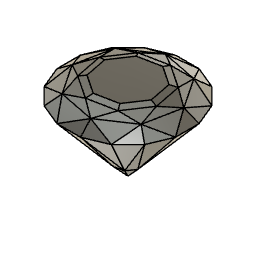
Diamond (Autodesk Fusion 360 design; units mm, degrees)
Autodesk Fusion 360 part; units mm, degrees
sketch "Sketch1" plane through (0, 0, 0) normal (0, 0, 1) x (1, 0, 0)
  line L0 (-3.5804, 18) -> (-10.1962, 15.2597)
  line L1 (-10.1962, 15.2597) -> (-15.2597, 10.1962)
  line L2 (-15.2597, 10.1962) -> (-18, 3.5804)
  line L3 (-18, 3.5804) -> (-18, -3.5804)
  line L4 (-18, -3.5804) -> (-15.2597, -10.1962)
  line L5 (-15.2597, -10.1962) -> (-10.1962, -15.2597)
  line L6 (-10.1962, -15.2597) -> (-3.5804, -18)
  line L7 (-3.5804, -18) -> (3.5804, -18)
  line L8 (3.5804, -18) -> (10.1962, -15.2597)
  line L9 (10.1962, -15.2597) -> (15.2597, -10.1962)
  line L10 (15.2597, -10.1962) -> (18, -3.5804)
  line L11 (18, -3.5804) -> (18, 3.5804)
  line L12 (18, 3.5804) -> (15.2597, 10.1962)
  line L13 (15.2597, 10.1962) -> (10.1962, 15.2597)
  line L14 (10.1962, 15.2597) -> (3.5804, 18)
  line L15 (3.5804, 18) -> (-3.5804, 18)
  dimension "d1" = 18
  measures "d1" distance of origin L15
extrude "Extrude1" add sketch "Sketch1" along normal blind 0 and the other way blind 17 draft -40
extrude "Extrude2" add 1 faces at (0.28, -1.4078, 0) along direction (0, 0, 1) blind 2.6 draft -56
sketch "Sketch2" plane through (0, 0, 2.6) normal (0, 0, 1) x (-1, 0, 0)
  line L0 (-8.0127, -11.9918) -> (-2.8137, -14.1453)
  line L1 (-2.8137, -14.1453) -> (2.8137, -14.1453)
  line L2 (2.8137, -14.1453) -> (8.0127, -11.9918)
  line L3 (8.0127, -11.9918) -> (11.9918, -8.0127)
  line L4 (11.9918, -8.0127) -> (14.1453, -2.8137)
  line L5 (14.1453, -2.8137) -> (14.1453, 2.8137)
  line L6 (14.1453, 2.8137) -> (11.9918, 8.0127)
  line L7 (11.9918, 8.0127) -> (8.0127, 11.9918)
  line L8 (8.0127, 11.9918) -> (2.8137, 14.1453)
  line L9 (2.8137, 14.1453) -> (-2.8137, 14.1453)
  line L10 (-2.8137, 14.1453) -> (-8.0127, 11.9918)
  line L11 (-8.0127, 11.9918) -> (-11.9918, 8.0127)
  line L12 (-11.9918, 8.0127) -> (-14.1453, 2.8137)
  line L13 (-14.1453, 2.8137) -> (-14.1453, -2.8137)
  line L14 (-14.1453, -2.8137) -> (-11.9918, -8.0127)
  line L15 (-11.9918, -8.0127) -> (-8.0127, -11.9918)
  line L16 (-2.8137, 14.1453) -> (-11.9918, 8.0127)
  line L17 (-10.1962, 15.2597, -2.6) -> (-2.8137, 14.1453, 0)
  line L18 (-10.1962, 15.2597, -2.6) -> (-11.9918, 8.0127, 0)
  point P0 (-10.1962, 15.2597)
  point P1 (-10.1962, 15.2597)
  constraint coincident L9.end L10.start
  constraint coincident L11.end L12.start
  constraint coincident P1 P0
extrude "Extrude3" cut sketch "Sketch2" along normal blind 1.5 contours L16 L17 L18 in plane through (1.5618, -2.3374, 8.0365) normal (0.255187, -0.381915, 0.888268)
pattern_circular "C-Pattern1" count 8 over 360 about axis through (0, 0, 1.75) along (0, 0, 1) of "Extrude3"
extrude "Extrude4" add 1 faces at (-0.9379, 4.7151, 2.6) along direction (0, 0, 1) blind 1.2 draft -62.7
sketch "Sketch3" plane through (0, 0, 3.8) normal (0, 0, 1) x (-1, 0, 0)
  line L0 (11.6772, 2.3227) -> (6.6146, 9.8994)
  line L1 (6.6146, 9.8994) -> (-2.3227, 11.6772)
  line L2 (-2.3227, 11.6772) -> (-9.8994, 6.6146)
  line L3 (-9.8994, 6.6146) -> (-11.6772, -2.3227)
  line L4 (-11.6772, -2.3227) -> (-6.6146, -9.8994)
  line L5 (-6.6146, -9.8994) -> (2.3227, -11.6772)
  line L6 (2.3227, -11.6772) -> (9.8994, -6.6146)
  line L7 (9.8994, -6.6146) -> (11.6772, 2.3227)
  line L8 (-6.1111, 9.1459) -> (-10.7883, 2.1459)
  line L9 (-10.7883, 2.1459, 0) -> (-11.9918, 8.0127, -1.2)
  line L10 (-11.9918, 8.0127, -1.2) -> (-6.1111, 9.1459, 0)
  point P0 (-11.9918, 8.0127)
  constraint midpoint L2 L8.start
  constraint midpoint L3 L8.end
extrude "Extrude5" cut sketch "Sketch3" along normal blind 4 contours L8 L9 L10 in plane through (0.6212, -0.415, 6.4521) normal (0.225438, -0.150633, 0.962542)
pattern_circular "C-Pattern2" count 8 over 360 about axis through (0, 0, 1.75) along (0, 0, 1) of 1 faces at (9.6304, -6.4348, 3.4)
extrude "Extrude6" add 1 faces at (0.2963, 1.4896, 3.8) along direction (0, 0, 1) blind 0.5 draft -75
sketch "Sketch4" plane through (0, 0, -17) normal (0, 0, -1) x (1, 0, 0)
  line L0 (-2.1159, -3.1666) -> (-0.743, -3.7353)
  line L1 (-0.743, -3.7353) -> (0.743, -3.7353)
  line L2 (0.743, -3.7353) -> (2.1159, -3.1666)
  line L3 (2.1159, -3.1666) -> (3.1666, -2.1159)
  line L4 (3.1666, -2.1159) -> (3.7353, -0.743)
  line L5 (3.7353, -0.743) -> (3.7353, 0.743)
  line L6 (3.7353, 0.743) -> (3.1666, 2.1159)
  line L7 (3.1666, 2.1159) -> (2.1159, 3.1666)
  line L8 (2.1159, 3.1666) -> (0.743, 3.7353)
  line L9 (0.743, 3.7353) -> (-0.743, 3.7353)
  line L10 (-0.743, 3.7353) -> (-2.1159, 3.1666)
  line L11 (-2.1159, 3.1666) -> (-3.1666, 2.1159)
  line L12 (-3.1666, 2.1159) -> (-3.7353, 0.743)
  line L13 (-3.7353, 0.743) -> (-3.7353, -0.743)
  line L14 (-3.7353, -0.743) -> (-3.1666, -2.1159)
  line L15 (-3.1666, -2.1159) -> (-2.1159, -3.1666)
  line L16 (-0.743, 3.7353) -> (2.1159, 3.1666)
  line L17 (2.1159, 3.1666, 0) -> (3.5804, 18, -17)
  line L18 (3.5804, 18, -17) -> (-0.743, 3.7353, 0)
  point P0 (3.5804, 18)
  constraint coincident L9.end L10.start
  constraint coincident L7.end L8.start
extrude "Extrude7" cut sketch "Sketch4" along normal blind 7 contours L16 L17 L18 in plane through (0.3897, -1.9592, -18.7431) normal (0.146996, -0.738997, -0.657476)
pattern_circular "C-Pattern3" count 8 over 360 about axis through (0, 0, 1.75) along (0, 0, 1) of "Extrude7"
extrude "Extrude8" add 1 faces at (-0.2477, -1.2451, -17) along direction (0, 0, -1) blind 5 draft -41.1
equation "d13 = 27.3 deg - 90 deg"
equation "d25 = 48.9 deg - 90 deg"
